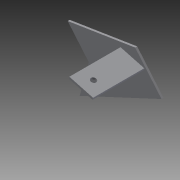
# Autodesk Inventor part: Left Bicep
Saved by Autodesk Inventor 2014 (Build 180170000, 170)
## iProperties
Created: 2015-08-01
Part Number: Left Bicep
Material: Generic
Document SubType Name: Modeling
Designer: Devon
Density: 1 g/cm^3
Appearance: Default
Author: Devon
Autodesk Inventor part; units mm, degrees
ref_plane "YZ Plane" through (0, 0, 0) normal (1, 0, 0) x (0, 1, 0)
ref_plane "XZ Plane" through (0, 0, 0) normal (0, 1, 0) x (-1, 0, 0)
ref_plane "XY Plane" through (0, 0, 0) normal (0, 0, 1) x (1, 0, 0)
sketch "Sketch1" plane through (0, 0, 0) normal (0, 0, 1) x (1, 0, 0)
  line L0 (-10.4788, 3.5567) -> (22.1748, -35.3584)
  line L1 (-10.4788, 3.5567) -> (40.3212, 3.5567) construction
  line L2 (22.1748, -35.3584) -> (8.205, -87.4942)
  line L3 (8.205, -87.4942) -> (134.8162, -28.4545)
  line L4 (134.8162, -28.4545) -> (93.9992, 20.1894)
  line L5 (93.9992, 20.1894) -> (-10.4788, 3.5567)
  point P0 (0, 0)
  dimension "d0" = 50.8
  dimension "d1" = 50
  dimension "d2" = 53.975
  dimension "d3" = 125
  dimension "d4" = 139.7
  dimension "d5" = 50
  dimension "d6" = 63.5
  dimension "d7" = 75
  constraints: 12 end point, 1 equal length, 1 horizontal, 1 parallel
  measures "d0" distance of L0.start L0.end
  measures "d1" angle of L0 L1
  measures "d2" distance of L0.end L2.end
  measures "d3" angle of L0 L2
  measures "d4" distance of L2.end L3.end
  measures "d5" angle of L3 L2
  measures "d6" distance of L3.end L4.end
  measures "d7" angle of L4 L3
extrude "Extrusion1" add sketch "Sketch1" along normal blind 3.175
sketch "Sketch2" plane through (0, 0, 3.175) normal (0, 0, 1) x (1, 0, 0)
  line L0 (22.1748, -35.3584) -> (8.205, -87.4942) projected
  line L1 (8.205, -87.4942) -> (8.205, -87.4942)
  line L2 (93.9992, 20.1894) -> (113.481, 20.1894) construction
  line L3 (88.957, 1.3714) -> (107.3579, -3.5591)
  line L4 (107.3579, -3.5591) -> (108.1796, -0.4923)
  line L5 (108.1796, -0.4923) -> (71.3778, 9.3687)
  line L6 (71.3778, 9.3687) -> (70.5561, 6.3019)
  line L7 (88.957, 1.3714) -> (70.5561, 6.3019)
  point P0 (0, 0)
  dimension "d10" = 19.4818
  dimension "d12" = 19.05
  dimension "d13" = 3.175
  dimension "d14" = 38.1
  constraints: 14 end point, 2 perpendicular, 1 collinear, 1 horizontal, 1 parallel, 1 point on line
  measures "d10" distance of L2.start L3.start
  measures "d12" distance of L3.start L3.end
  measures "d13" distance of L3.end L4.end
  measures "d14" distance of L4.end L5.end
extrude "Extrusion2" add sketch "Sketch2" along normal blind 79.2734
sketch "Sketch3" plane through (71.3778, 9.3687, 82.4484) normal (0.2588, 0.9659, 0) x (0.9659, -0.2588, 0)
  line L0 (0, 0) -> (19.05, 0)
  line L1 (19.05, 0) -> (19.05, 19.05)
  line L2 (19.05, 19.05) -> (0, 19.05)
  line L3 (0, 19.05) -> (0, 0)
  point P0 (-66.5209, 82.4484)
  dimension "d17" = 19.05
  dimension "d18" = 19.05
  constraints: 8 end point, 2 parallel, 1 horizontal, 1 perpendicular
  measures "d17" distance of L2.end L1.end
  measures "d18" distance of L1.end L0.end
hole "Hole1" at (89.7787, 4.4382, 63.3984) direction (-0.2588, -0.9659, 0) diameter 8.3312 end through all
body "Solid1"
